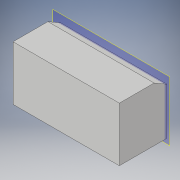
# Autodesk Inventor part: Part1
Saved by Autodesk Inventor 2017 (Build 210142000, 142)
## iProperties
Created: 2019-08-05
Part Number: Part1
Material: Generic
Document SubType Name: Modeling
Designer: user
Density: 1 g/cm^3
Appearance: Default
Author: user
Autodesk Inventor part; units mm, degrees
ref_plane "YZ Plane" through (0, 0, 0) normal (1, 0, 0) x (0, 1, 0)
ref_plane "XZ Plane" through (0, 0, 0) normal (0, 1, 0) x (-1, 0, 0)
ref_plane "XY Plane" through (0, 0, 0) normal (0, 0, 1) x (1, 0, 0)
sketch "Sketch1" plane through (0, 0, 0) normal (1, 0, 0) x (0, 1, 0)
  point P0 (0, 0)
sketch "Sketch2" plane through (0, 0, 0) normal (1, 0, 0) x (0, 1, 0)
  line L0 (-127.5, -112) -> (127.5, -112)
  line L1 (127.5, -112) -> (127.5, 112)
  line L2 (127.5, 112) -> (-127.5, 112)
  line L3 (-127.5, 112) -> (-127.5, -112)
  line L4 (-127.5, -112) -> (127.5, 112) construction
  line L5 (127.5, -112) -> (-127.5, 112) construction
  line L6 (127.5, -52) -> (92.5, -112)
  point P0 (0, 0)
  dimension "d0" = 255
  dimension "d1" = 224
  dimension "d2" = 35
  dimension "d3" = 60
  constraints: 14 end point, 2 midpoint, 2 parallel, 2 point on line, 1 horizontal, 1 perpendicular
  measures "d0" distance of L2.end L1.end
  measures "d1" distance of L1.end L0.end
  measures "d2" distance of L6.end L0.end
  measures "d3" distance of L0.end L6.start
extrude "Extrusion1" add sketch "Sketch2" along normal blind 500 contours L3 L2 L1 L6 L0
shell "Shell1" thickness 22.5 removed faces 0
ref_plane "Work Plane1" through (0, -127.5, -100.75) normal (0, 0, -1) x (-1, 0, 0)
sketch "Sketch3" plane through (0, -127.5, -112) normal (0, 0, -1) x (-1, 0, 0)
  line L0 (-105.6, 103) -> (-190.4, 103)
  line L1 (-190.4, 103) -> (-190.4, 129.4)
  line L2 (-190.4, 129.4) -> (-105.6, 129.4)
  line L3 (-105.6, 129.4) -> (-105.6, 103)
  point P0 (0, 127.5)
  dimension "d7" = 84.8
  dimension "d8" = 26.4
  constraints: 8 end point, 2 parallel, 1 horizontal, 1 perpendicular
  measures "d7" distance of L1.end L2.end
  measures "d8" distance of L0.end L1.end
extrude "Extrusion2" cut sketch "Sketch3" against normal blind 201.5
sketch "Sketch4" plane through (0, -127.5, -112) normal (0, 0, -1) x (-1, 0, 0)
  line L0 (-269.6, 140.8) -> (-320.36, 140.8)
  line L1 (-320.36, 140.8) -> (-320.36, 90.04)
  line L2 (-320.36, 90.04) -> (-269.6, 90.04)
  line L3 (-269.6, 90.04) -> (-269.6, 140.8)
  line L4 (0, 220) -> (-500, 220) projected
  line L5 (-190.4, 103) -> (-190.4, 129.4) projected
  point P0 (0, 127.5)
  dimension "d11" = 50.76
  dimension "d12" = 50.76
  dimension "d13" = 79.2
  dimension "d14" = 79.2
  constraints: 8 end point, 2 parallel, 1 horizontal, 1 perpendicular
  measures "d11" distance of L2.end L1.end
  measures "d12" distance of L1.end L0.end
  measures "d13" distance between parallel lines of L0 L4
  measures "d14" distance between parallel lines of L5 L3
extrude "Extrusion3" cut sketch "Sketch4" against normal blind 201.5
body "Solid1"
